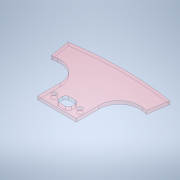
# Autodesk Inventor part: sensor
Saved by Autodesk Inventor 2022 (Build 260153000, 153)
## iProperties
Created: 2021-10-17
Part Number: sensor
Material: エポキシ樹脂
Document SubType Name: Modeling
Designer: shiok
Density: 1.14 g/cm^3
Appearance: 透明 - スレート 青
Mass: 1.6944 g
Surface Area: 21.5521 cm^2
Volume: 1.48632 cm^3
Author: shiok
Autodesk Inventor part; units mm, degrees
note: some values were not read from the file. Chosen so that the rebuilt part matches the saved one: direction of "穴1".
ref_plane "YZ Plane" through (0, 0, 0) normal (1, 0, 0) x (0, 1, 0)
ref_plane "XZ Plane" through (0, 0, 0) normal (0, 1, 0) x (-1, 0, 0)
ref_plane "XY Plane" through (0, 0, 0) normal (0, 0, 1) x (1, 0, 0)
sketch "スケッチ1" plane through (0, 0, 0) normal (0, 1, 0) x (-1, 0, 0)
  arc A0 (0, -155) -> (25, -152.9706) centre (0, 0) ccw
  line L0 (25, -152.9706) -> (0, 0)
  line L1 (0, 0) -> (0, -144.6885)
  arc A1 (9.5, -144.6885) -> (23.3871, -143.1015) centre (0, 0) ccw
  line L2 (9.5, -144.6885) -> (9.5, -122.5)
  line L3 (9.5, -122.5) -> (0, -122.5)
  arc A2 (-25, -152.9706) -> (0, -155) centre (0, 0) ccw
  line L4 (-25, -152.9706) -> (0, 0)
  arc A3 (-23.3871, -143.1015) -> (-9.5, -144.6885) centre (0, 0) ccw
  line L5 (-9.5, -144.6885) -> (-9.5, -122.5)
  line L6 (-9.5, -122.5) -> (0, -122.5)
  line L7 (9.5, -144.6885) -> (0, -144.6885) construction
  line L8 (-9.5, -144.6885) -> (0, -144.6885) construction
  line L9 (-9.5, -180.2611) -> (-9.5, 6.4286)
  line L10 (9.5, -180.2611) -> (9.5, 6.4286)
  line L11 (0, -130) -> (-3.1667, -130)
  line L12 (-3.1667, -130) -> (-3.1667, -125)
  line L13 (-3.1667, -125) -> (0, -125)
  line L14 (0, -130) -> (3.1667, -130)
  line L15 (3.1667, -130) -> (3.1667, -125)
  line L16 (3.1667, -125) -> (0, -125)
  line L17 (0, -144.6885) -> (0, -145)
  line L18 (0, -145) -> (0, -155)
  point P0 (0, -125)
  point P1 (0, -150)
  dimension "d4" = 19
  dimension "d12" = 122.5
  dimension "d13" = 10
  dimension "d29" = 19
  dimension "d32" = 5
  dimension "d33" = 6.3333
  dimension "d34" = 2.5
  dimension "d36" = 50
  dimension "d38" = 150
  constraints: 38 end point, 9 point on circle, 8 symmetric about line, 7 perpendicular, 7 point on line, 4 centre point, 4 coincident, 4 vertical, 2 midpoint, 1 horizontal, 1 parallel, 2 other
  measures "d4" distance of L2.end L5.end
  measures "d12" distance from line of point (0, 0) L3
  measures "d13" radial gap between concentric circles of A0 A1
  measures "d29" distance between parallel lines of L9 L10
  measures "d32" distance of L11.end L12.end
  measures "d33" distance between parallel lines of L15 L12
  measures "d34" distance between parallel lines of L13 L6
  measures "d36" distance of L4.start L0.start
  measures "d38" distance of point (0, 0) point (0, -150)
extrude "押し出し1" add sketch "スケッチ1" along normal blind 1.6 contours L18 L17 L1 L14 L15 L16 L3 L2 L10 A0 | A2 L9 L5 L6 L1 L13 L12 L11 L17 L18 | L10 A1 L0 A0 | A2 L4 A3 L9
sketch "スケッチ2" plane through (0, 1.6, 0) normal (0, 1, 0) x (1, 0, 0)
  line L0 (9.5, 122.5) -> (9.5, 144.6885) projected
  arc A0 (23.3871, 143.1015) -> (9.5, 144.6885) centre (0, 0) ccw projected
  line L1 (23.3871, 143.1015) -> (25, 152.9706) projected
  arc A1 (25, 152.9706) -> (-25, 152.9706) centre (0, 0) ccw projected
  line L2 (-25, 152.9706) -> (-23.3871, 143.1015) projected
  arc A2 (-9.5, 144.6885) -> (-23.3871, 143.1015) centre (0, 0) ccw projected
  line L3 (-9.5, 144.6885) -> (-9.5, 122.5) projected
  line L4 (-9.5, 122.5) -> (9.5, 122.5) projected
  line L5 (-9.5, 122.5) -> (5.5, 122.5)
  line L6 (5.5, 122.5) -> (5.5, 132.5)
  line L7 (5.5, 132.5) -> (-9.5, 132.5)
  line L8 (-9.5, 132.5) -> (-9.5, 122.5)
  line L9 (-6.3333, 127.5) -> (-3.1667, 127.5) construction
  line L10 (-6.3333, 127.5) -> (-9.5, 127.5) construction
  line L11 (-3.1667, 125) -> (-3.1667, 130) projected
  point P0 (6.3333, 127.5)
  dimension "d19" = 10
  dimension "d20" = 15
  constraints: 12 end point, 2 collinear, 2 parallel, 1 horizontal, 1 midpoint, 1 perpendicular, 2 other
  measures "d19" distance of L6.end L5.end
  measures "d20" distance of L6.end L7.end
hole "穴1" at (6.3333, 1.6, -127.5) at (-6.3333, 1.6, -127.5) direction (0, -1, 0) diameter 2.4 depth 1.6 clearance for "Countersunk Flat Head Screw ISO 2009/7046" size "M2" standard "ISO"
fillet "フィレット1" radius 10 2 edges at (9.5, 0.8, -144.6885) (-9.5, 0.8, -144.6885)
fillet "フィレット2" radius 1.5 4 edges at (-3.1667, 0.8, -130) (3.1667, 0.8, -125) (3.1667, 0.8, -130) (-3.1667, 0.8, -125)
